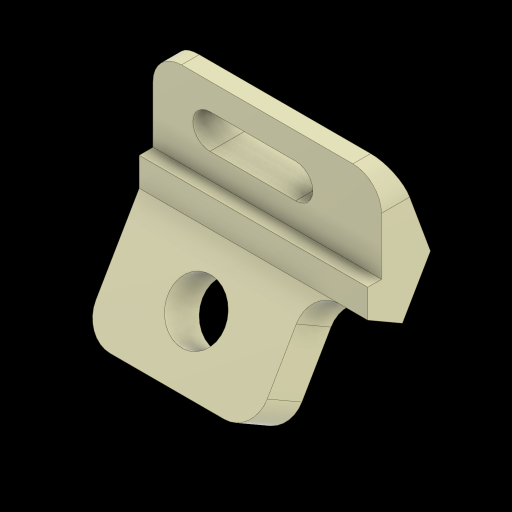
# Autodesk Inventor part: ANS9-2-BK
Saved by Autodesk Inventor 2024 (Build 280153000, 153)
## iProperties
Created: 2023-10-29
Part Number: ANS9-2-BK
Material: Polypropylene
Document SubType Name: Modeling
Designer: bennk
Density: 0.899 g/cm^3
Appearance: Smooth - Ash
Mass: 16.3778 g
Surface Area: 66.7691 cm^2
Volume: 18.2178 cm^3
Author: bennk
Autodesk Inventor part; units mm, degrees
ref_plane "YZ Plane" through (0, 0, 0) normal (1, 0, 0) x (0, 1, 0)
ref_plane "XZ Plane" through (0, 0, 0) normal (0, 1, 0) x (-1, 0, 0)
ref_plane "XY Plane" through (0, 0, 0) normal (0, 0, 1) x (1, 0, 0)
sketch "Sketch1" plane through (0, 0, 0) normal (1, 0, 0) x (0, 1, 0)
  line L0 (0, 0) -> (-32.9956, 19.05)
  line L1 (-32.9956, 19.05) -> (-28.5506, 26.749)
  line L2 (-28.5506, 26.749) -> (-6.35, 13.9315)
  line L3 (-6.35, 13.9315) -> (0, 13.9315)
  line L4 (0, 13.9315) -> (0, 10.8835)
  line L5 (0, 10.8835) -> (19.05, 10.8835)
  line L6 (19.05, 10.8835) -> (19.05, 6.9336)
  line L7 (19.05, 6.9336) -> (0, 0)
  dimension "d0" = 38.1
  dimension "d1" = 8.89
  dimension "d2" = 30
  dimension "d3" = 19.05
  dimension "d5" = 3.048
  dimension "d6" = 20
  dimension "d7" = 6.35
  constraints: 16 end point, 4 perpendicular, 1 horizontal, 1 point on line, 1 vertical
  measures "d0" distance of L0.start L0.end
  measures "d1" distance of L0.end L1.end
  measures "d2" angle of L3 L2
  measures "d3" distance of L4.end L5.end
  measures "d5" distance of L3.end L4.end
  measures "d6" angle of L7 L5
  measures "d7" distance of L2.end L3.end
extrude "MAIN BODY" add sketch "Sketch1" along normal blind 50.8
sketch "Sketch2" plane through (0, 0, 10.8835) normal (0, 0, 1) x (1, 0, 0)
  line L0 (12.7, 9.398) -> (31.75, 9.398) construction
  line L1 (12.7, 5.588) -> (31.75, 5.588)
  line L2 (31.75, 13.208) -> (12.7, 13.208)
  arc A0 (12.7, 13.208) -> (12.7, 5.588) centre (12.7, 9.398) ccw
  arc A1 (31.75, 5.588) -> (31.75, 13.208) centre (31.75, 9.398) ccw
  line L3 (0, 19.05) -> (0, 0) projected
  line L4 (0, 19.05) -> (50.8, 19.05) projected
  line L5 (0, 0) -> (50.8, 0) projected
  point P0 (22.225, 9.398)
  dimension "d11" = 7.62
  dimension "d12" = 19.05
  dimension "d13" = 12.7
  dimension "d15" = 9.398
  constraints: 8 end point, 4 point on circle, 4 tangent, 2 centre point, 1 horizontal, 1 midpoint, 1 parallel
  measures "d11" diameter of A1
  measures "d12" distance of L2.start L2.end
  measures "d13" distance from line of L3 L0.start
  measures "d15" distance from line of L5 L0.start
extrude "SLOT CUTOUT" cut sketch "Sketch2" against normal through all
sketch "Sketch3" plane through (0, -28.5506, 26.749) normal (0, 0.5, 0.8660254) x (1, 0, 0)
  circle A0 centre (19.05, 12.935) radius 6.35
  line L0 (38.1, 25.635) -> (50.8, 25.635)
  line L1 (50.8, 25.635) -> (50.8, 0)
  line L2 (50.8, 0) -> (38.1, 0)
  line L3 (38.1, 0) -> (38.1, 25.635)
  line L4 (0, 25.635) -> (0, 0) projected
  line L5 (0, 25.635) -> (50.8, 25.635) projected
  line L6 (50.8, 25.635) -> (50.8, 0) projected
  line L7 (0, 0) -> (50.8, 0) projected
  point P0 (0, 38.1)
  dimension "d18" = 12.7
  dimension "d19" = 19.05
  dimension "d20" = 12.7
  dimension "d21" = 38.1
  constraints: 8 end point, 3 collinear, 2 parallel, 1 centre point, 1 horizontal, 1 perpendicular
  measures "d18" diameter of A0
  measures "d19" distance from line of L4 A0.centre
  measures "d20" distance from line of L5 A0.centre
  measures "d21" distance between parallel lines of L4 L3
extrude "CIRC AND RECT CUTOUT" cut sketch "Sketch3" against normal through all contours A0 | L0 L1 L2 L3
fillet ".25 filliets" radius 6.35 5 edges at (50.8, 19.05, 8.9085) (0, 19.05, 8.9085) (38.1, -8.5725, 10.082) (38.1, -30.7731, 22.8995) (0, -30.7731, 22.8995)
body "Solid1"
